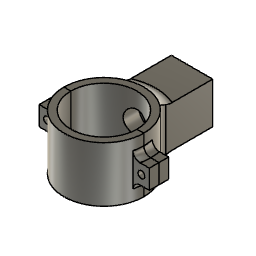
RAMSES_holder v6 (Autodesk Fusion 360 design; units mm, degrees)
Autodesk Fusion 360 part; units mm, degrees
sketch "Sketch1" plane through (0, 0, 0) normal (0, 1, 0) x (1, 0, 0)
  line L0 (-8, 5.2993) -> (-6.6428, 5.2993)
  line L1 (3.44, 4.5007) -> (-3.44, 4.5007)
  line L2 (-3.44, -4.5007) -> (3.44, -4.5007)
  circle A0 centre (0, 0) radius 2.5
  line L3 (3.3572, -4.7007) -> (5.2993, -6.6428)
  line L4 (-8.2, -5.4993) -> (-8.2, -2.84)
  line L5 (8, -5.2993) -> (6.6428, -5.2993)
  line L6 (10.2, -4.5572) -> (10.2, -2.3572)
  line L7 (-2.3572, -10.2) -> (-4.5572, -10.2)
  line L8 (10.2, -4.5572) -> (8, -2.3572)
  line L9 (-4.5572, -10.2) -> (-2.3572, -8)
  line L10 (2.3572, -8) -> (4.5572, -10.2)
  line L11 (-2.3572, -8) -> (-2.3572, -10.2)
  line L12 (-10.2, -4.5572) -> (-10.2, -10.2)
  line L13 (-2.3572, -8) -> (-5.2993, -8)
  line L14 (-10, -4.64) -> (-10, -10)
  line L15 (-5.2993, -8) -> (-5.2993, -6.6428)
  line L16 (4.5572, -10.2) -> (2.3572, -10.2)
  line L17 (-8, -2.3572) -> (-10.2, -4.5572)
  line L18 (10.2, -10.2) -> (10.2, -4.5572)
  line L19 (-4.7007, -3.3572) -> (-6.6428, -5.2993)
  line L20 (-10.2, -2.3572) -> (-10.2, -4.5572)
  line L21 (-2.84, 8.2) -> (-4.64, 10)
  line L22 (5.2993, -6.6428) -> (5.2993, -8)
  line L23 (5.2993, -8) -> (2.3572, -8)
  line L24 (-8, -2.3572) -> (-10.2, -2.3572)
  line L25 (10.2, -2.3572) -> (8, -2.3572)
  line L26 (-6.6428, -5.2993) -> (-8, -5.2993)
  line L27 (6.6428, -5.2993) -> (4.7007, -3.3572)
  line L28 (5.4993, -8.2) -> (2.84, -8.2)
  line L29 (5.4993, -6.56) -> (5.4993, -8.2)
  line L30 (-10, -10) -> (-4.64, -10)
  line L31 (-6.56, -5.4993) -> (-8.2, -5.4993)
  line L32 (-8.2, -2.84) -> (-10, -4.64)
  line L33 (-4.64, 10) -> (-10, 10)
  line L34 (-4.5007, -3.44) -> (-6.56, -5.4993)
  line L35 (-8, -5.2993) -> (-8, -2.3572)
  line L36 (-4.64, -10) -> (-2.84, -8.2)
  line L37 (-5.4993, -8.2) -> (-5.4993, -6.56)
  line L38 (3.44, -4.5007) -> (5.4993, -6.56)
  line L39 (4.5572, -10.2) -> (10.2, -10.2)
  line L40 (-5.4993, -6.56) -> (-3.44, -4.5007)
  line L41 (8, -2.3572) -> (8, -5.2993)
  line L42 (-3.3572, 4.7007) -> (-5.2993, 6.6428)
  line L43 (-3.3572, -4.7007) -> (3.3572, -4.7007)
  line L44 (2.84, -8.2) -> (4.64, -10)
  line L45 (8, 5.2993) -> (8, 2.3572)
  line L46 (-6.6428, 5.2993) -> (-4.7007, 3.3572)
  line L47 (3.3572, 4.7007) -> (-3.3572, 4.7007)
  line L48 (4.5572, 10.2) -> (2.3572, 8)
  line L49 (-5.4993, 8.2) -> (-2.84, 8.2)
  line L50 (-10.2, 2.3572) -> (-10.2, 4.5572)
  line L51 (4.64, -10) -> (10, -10)
  line L52 (10, -10) -> (10, -4.64)
  line L53 (-2.84, -8.2) -> (-5.4993, -8.2)
  line L54 (-10.2, -10.2) -> (-4.5572, -10.2)
  line L55 (-5.2993, -6.6428) -> (-3.3572, -4.7007)
  line L56 (8.2, 2.84) -> (10, 4.64)
  line L57 (-8, 2.3572) -> (-8, 5.2993)
  line L58 (-4.5572, 10.2) -> (-10.2, 10.2)
  line L59 (8.2, -2.84) -> (8.2, -5.4993)
  line L60 (-8.2, 2.84) -> (-8.2, 5.4993)
  line L61 (10, -4.64) -> (8.2, -2.84)
  line L62 (-10, 10) -> (-10, 4.64)
  line L63 (-10, 4.64) -> (-8.2, 2.84)
  line L64 (10, 10) -> (4.64, 10)
  line L65 (10, 4.64) -> (10, 10)
  line L66 (5.2993, 6.6428) -> (3.3572, 4.7007)
  line L67 (-10.2, 10.2) -> (-10.2, 4.5572)
  line L68 (-8, 2.3572) -> (-10.2, 2.3572)
  line L69 (4.5007, 3.44) -> (6.56, 5.4993)
  line L70 (-5.2993, 8) -> (-2.3572, 8)
  line L71 (8, 2.3572) -> (10.2, 4.5572)
  line L72 (-5.2993, 6.6428) -> (-5.2993, 8)
  line L73 (4.7007, -3.3572) -> (4.7007, 3.3572)
  line L74 (-4.7007, 3.3572) -> (-4.7007, -3.3572)
  line L75 (10.2, 4.5572) -> (10.2, 10.2)
  line L76 (5.2993, 8) -> (5.2993, 6.6428)
  line L77 (8, 2.3572) -> (10.2, 2.3572)
  line L78 (-2.3572, 10.2) -> (-2.3572, 8)
  line L79 (6.6428, 5.2993) -> (8, 5.2993)
  line L80 (-4.5572, 10.2) -> (-2.3572, 10.2)
  line L81 (2.3572, 8) -> (5.2993, 8)
  line L82 (4.7007, 3.3572) -> (6.6428, 5.2993)
  line L83 (-8.2, 5.4993) -> (-6.56, 5.4993)
  line L84 (2.3572, 10.2) -> (4.5572, 10.2)
  line L85 (4.64, 10) -> (2.84, 8.2)
  line L86 (6.56, 5.4993) -> (8.2, 5.4993)
  line L87 (8.2, 5.4993) -> (8.2, 2.84)
  line L88 (6.56, -5.4993) -> (4.5007, -3.44)
  line L89 (-5.4993, 6.56) -> (-5.4993, 8.2)
  line L90 (5.4993, 6.56) -> (3.44, 4.5007)
  line L91 (-10.2, 4.5572) -> (-8, 2.3572)
  line L92 (-4.5007, 3.44) -> (-4.5007, -3.44)
  line L93 (4.5007, -3.44) -> (4.5007, 3.44)
  line L94 (-6.56, 5.4993) -> (-4.5007, 3.44)
  line L95 (5.4993, 8.2) -> (5.4993, 6.56)
  line L96 (2.3572, -10.2) -> (2.3572, -8)
  line L97 (-2.3572, 8) -> (-4.5572, 10.2)
  line L98 (10.2, 10.2) -> (4.5572, 10.2)
  line L99 (10.2, 2.3572) -> (10.2, 4.5572)
  line L100 (2.84, 8.2) -> (5.4993, 8.2)
  line L101 (2.3572, 8) -> (2.3572, 10.2)
  line L102 (8.2, -5.4993) -> (6.56, -5.4993)
  line L103 (-3.44, 4.5007) -> (-5.4993, 6.56)
  line L104 (15, 15) -> (-15, 15)
  line L105 (-15, 15) -> (-15, -15)
  line L106 (-15, -15) -> (15, -15)
  line L107 (15, -15) -> (15, 15)
  line L108 (15, 15) -> (-15, -15) construction
  line L109 (-15, 15) -> (15, -15) construction
  dimension "d143" = 0.2
  dimension "d2" = 30
  dimension "d3" = 30
  dimension "d13" = 5
  constraint parallel L70 L80
  constraint perpendicular L70 L78
  constraint perpendicular L67 L68
  constraint perpendicular L50 L68
  constraint perpendicular L81 L101
  constraint perpendicular L84 L101
  constraint perpendicular L75 L77
  constraint perpendicular L77 L99
  constraint parallel L6 L18
  constraint perpendicular L18 L25
  constraint parallel L16 L39
  constraint perpendicular L23 L96
  constraint perpendicular L11 L54
  constraint perpendicular L7 L11
  constraint perpendicular L12 L24
  constraint perpendicular L20 L24
  constraint horizontal L104
  constraint perpendicular L104 L105
  constraint parallel L104 L106
  constraint parallel L105 L107
  constraint coincident L108 A0.centre
  constraint coincident L109 A0.centre
  constraint coincident A0.centre origin
  measures "d2" distance of L105.end L106.end
  measures "d3" distance of L104.end L105.end
  measures "d13" diameter of A0
extrude "Extrude1" add sketch "Sketch1" along normal blind 25 contours L104 L105 L106 L107 makes body 1
extrude "Extrude2" add sketch "Sketch1" against normal blind 5 contours L0 L3 L5 L8 L9 L10 L12 L13 L15 L17 L18 L19 L22 L23 L26 L27 L35 L39 L41 L42 L43 L45 L46 L47 L48 L54 L55 L57 L58 L66 L67 L70 L71 L72 L73 L74 L75 L76 L79 L81 L82 L91 L97 L98 | L50 L68 L91 | L78 L80 L97 | L17 L20 L24 | L7 L9 L11 | L48 L84 L101 | L71 L77 L99 | L10 L16 L96 | L6 L8 L25 | L1 L2 L4 L14 L21 L28 L29 L30 L31 L32 L33 L34 L36 L37 L38 L40 L44 L49 L51 L52 L53 L56 L59 L60 L61 L62 L63 L64 L65 L69 L83 L85 L86 L87 L88 L89 L90 L92 L93 L94 L95 L100 L102 L103 | L104 L105 L106 L107 bodies 1
sketch "Sketch2" plane through (0, 0, 0) normal (0, 0, 1) x (1, 0, 0)
  line L0 (15, -5) -> (15, 25)
  line L1 (15, 25) -> (-15, 25)
  line L2 (-15, 25) -> (-15, -5)
  line L3 (-15, -5) -> (15, -5)
  line L4 (0, -5) -> (0, -15)
  line L5 (0, -15) -> (0, -39)
  circle A0 centre (0, -39) radius 24
  circle A1 centre (0, -39) radius 29
  line L6 (40, -46) -> (-40, -46)
  line L7 (-40, -46) -> (-40, -32)
  line L8 (-40, -32) -> (40, -32)
  line L9 (40, -32) -> (40, -46)
  line L10 (40, -46) -> (-40, -32) construction
  line L11 (-40, -46) -> (40, -32) construction
  point P0 (0, -39)
  dimension "d8" = 10
  dimension "d9" = 24
  dimension "d10" = 80
  dimension "d11" = 14
  constraint midpoint L3 L4.start
  constraint perpendicular L3 L4
  constraint vertical L5
  constraint coincident P0 L5.end
  constraint coincident L4.end A0
  constraint horizontal L6
  constraint perpendicular L6 L7
  constraint parallel L6 L8
  constraint parallel L7 L9
  constraint coincident L10 P0
  constraint coincident L11 P0
  measures "d8" distance of L4.start L4.end
  measures "d9" distance of L4.end P0
  measures "d10" distance of L7.end L8.end
  measures "d11" distance of L6.end L7.end
sketch "Sketch3" plane through (0, -5, 0) normal (0, -1, 0) x (1, 0, 0)
  circle A0 centre (0, 0) radius 2.5
  line L0 (15, -15) -> (15, 15)
  line L1 (15, 15) -> (-15, 15)
  line L2 (-15, 15) -> (-15, -15)
  line L3 (-15, -15) -> (15, -15)
  circle A1 centre (0, 0) radius 8.5
  dimension "d12" = 17
  constraint coincident A0.centre A1.centre
  measures "d12" diameter of A1
extrude "Extrude3" add sketch "Sketch2" along normal mid plane 40 separate body contours L4 A0 A1 L8 | L4 A0 A1 L8 | A0 A1 L6 L8 | A0 A1 L6 L8 | A0 A1 L6 makes body 2
extrude "Extrude4" add sketch "Sketch2" along normal mid plane 14 contours A1 L6 L8 L9 | A1 L6 L7 L8 bodies 2
extrude "Extrude5" add sketch "Sketch3" along normal up to surface contours L0 L1 L2 L3 end surface at (26.9263, -49.7691, -2.3333) on bodies 2 bodies 1 2
extrude "Extrude6" cut sketch "Sketch3" along normal blind 27 contours A0 | A1 bodies 1
sketch "Sketch4" plane through (0, -46, 0) normal (0, -1, 0) x (1, 0, 0)
  line L0 (-28.1425, -7) -> (-28.1425, 7)
  line L1 (-28.1425, 7) -> (-40, 7)
  line L2 (-40, 7) -> (-40, -7)
  line L3 (-40, -7) -> (-28.1425, -7)
  line L4 (40, -7) -> (40, 7)
  line L5 (40, 7) -> (28.1425, 7)
  line L6 (28.1425, 7) -> (28.1425, -7)
  line L7 (28.1425, -7) -> (40, -7)
  line L8 (-29.7829, 2.5981) -> (-34.2829, 5.1962)
  line L9 (-34.2829, 5.1962) -> (-38.7829, 2.5981)
  line L10 (-38.7829, 2.5981) -> (-38.7829, -2.5981)
  line L11 (-38.7829, -2.5981) -> (-34.2829, -5.1962)
  line L12 (-34.2829, -5.1962) -> (-29.7829, -2.5981)
  line L13 (-29.7829, -2.5981) -> (-29.7829, 2.5981)
  line L14 (38.7017, 2.5981) -> (34.2017, 5.1962)
  line L15 (34.2017, 5.1962) -> (29.7017, 2.5981)
  line L16 (29.7017, 2.5981) -> (29.7017, -2.5981)
  line L17 (29.7017, -2.5981) -> (34.2017, -5.1962)
  line L18 (34.2017, -5.1962) -> (38.7017, -2.5981)
  line L19 (38.7017, -2.5981) -> (38.7017, 2.5981)
  line L20 (40, 0) -> (-40, 0)
  circle A0 centre (-34.2829, 0) radius 2.5
  circle A1 centre (34.2017, 0) radius 2.5
  point P0 (-34.2829, 0)
  point P1 (34.2017, 0)
  dimension "d22" = 4.5
  dimension "d23" = 4.5
  dimension "d26" = 5
  dimension "d27" = 5
  constraint coincident P1 L20
  constraint coincident P0 A0.centre
  constraint coincident P1 A1.centre
  measures "d22" distance of P0 L13
  measures "d23" distance of P1 L19
  measures "d26" diameter of A0
  measures "d27" diameter of A1
extrude "Extrude7" cut sketch "Sketch4" along normal blind 2 from surface at -14 contours L8 L9 L10 L13 L20 A0 | L10 L11 L12 L13 L20 A0 | L20 A0 | L20 A0 | L14 L15 L16 L19 L20 A1 | L16 L17 L18 L19 L20 A1 | L20 A1 | L20 A1 bodies 1
extrude "Extrude8" cut sketch "Sketch4" against normal blind 36 contours L20 A0 | L20 A0 | L20 A1 | L20 A1 bodies 1
ref_plane "WorkPlane1" through (34.0712, -39, 0) normal (0, 1, 0) x (-1, 0, 0)
fillet "Fillet1" radius 5 4 edges at (29, -39, 7) (29, -39, -7) (-29, -39, 7) (-29, -39, -7) on bodies 1
fillet "Fillet2" radius 10 4 edges at (-15, -14.1807, 0) (15, -14.1807, 0) (0, -10, 15) (0, -10, -15) on bodies 1
split "Split1" by plane through (34.0712, -39, 0) normal (0, 1, 0) bodies 1 makes body 3 at (-10.8629, -17.5991, 0.0687)
